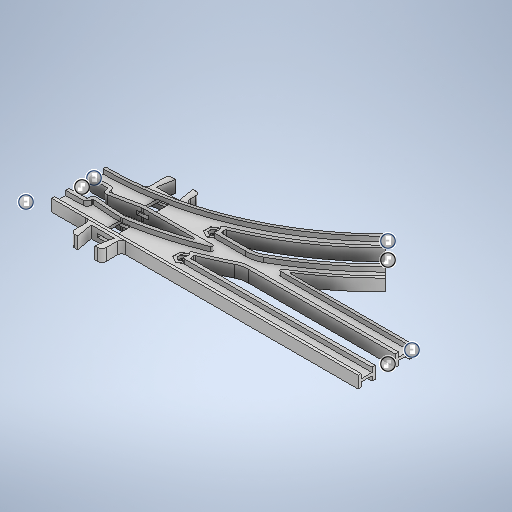
# Autodesk Inventor part: RR_SingleTurnout-all
Saved by Autodesk Inventor 2025.1 (Build 291241000, 241)
## iProperties
Created: 2025-03-05
Part Number: RR_SingleTurnout-all
Material: 一般
Document SubType Name: Modeling
Designer: kumagai
Density: 1 g/cm^3
Appearance: 既定
d0: 244.000 mm
d1: 10.000 mm
d2: 215.000 mm
d3: 5.000 mm
d4: 38.000 mm
d5: 18.600 mm
d6: 2.000 mm
d7: 2.400 mm
d8: 215.000 mm
d9: 45.00 deg
d11: 15.000 mm
d12: 15.000 mm
d13: 2.000 mm
d14: 0.00 deg
d15: 8.400 mm
d16: 0.00 deg
d17: 0.500 mm
d18: 1.000 mm
d19: 20.000 mm
d20: 20.000 mm
d21: 0.500 mm
d22: 1.000 mm
d23: 3.000 mm
d26: 3.000 mm
d27: 3.500 mm
d28: 2.400 mm
d29: 1.000 mm
d30: 5.000 mm
d32: 3.000 mm
d33: 3.000 mm
d34: 3.500 mm
d35: 2.400 mm
d36: 3.000 mm
d37: 1.000 mm
d38: 5.000 mm
d39: 19.000 mm
d41: 0.000 mm
d42: 0.000 mm
d43: 0.000 mm
d44: 0.000 mm
d45: 0.000 mm
d46: 0.000 mm
d47: 0.000 mm
d48: 0.000 mm
d49: 0.000 mm
d51: 6.000 mm
d52: 10.700 mm
d53: 0.300 mm
d55: 2.400 mm
d56: 10.000 mm
d57: 6.000 mm
d58: 0.300 mm
d59: 2.000 mm
d60: 5.000 mm
d62: 2.400 mm
d63: 1.200 mm
d65: 1.200 mm
d66: 41.500 mm
d67: 36.900 mm
TurnoutRadius: 215.000 mm
d40: 19.000 mm
d50: 10.700 mm
PrinterOffset: 0.000 mm
StraightLength: 215.000 mm
RailWidth: 38.000 mm
OuterWall: 2.000 mm
InnerWall: 2.400 mm
InsideWidth: 18.600 mm
RailHeight: 8.400 mm
RailDepth: 3.200 mm
ConnectorLength: 15.000 mm
JointMW1: 13.000 mm
JointMW2: 9.400 mm
JointMH: 9.000 mm
JointFW1: 13.300 mm
JointFW2: 9.600 mm
JointFH: 9.500 mm
DoubleWidth: 60.000 mm
ViaductHeight: 66.000 mm
SupportGap: 0.200 mm
SupportRib: 0.650 mm
JointRadius: 12.000 mm
JointRSLength: 15.000 mm
JointRSTP: 3.000 mm
RailThick: 2.000 mm
Author: kumagai
Autodesk Inventor part; units mm, degrees
ref_plane "YZ Plane" through (0, 0, 0) normal (1, 0, 0) x (0, 1, 0)
ref_plane "XY Plane" through (0, 0, 0) normal (0, 0, 1) x (1, 0, 0)
sketch "MainSketch" plane through (0, 0, 0) normal (0, 1, 0) x (-1, 0, 0)
  line L0 (0, -306.5136) -> (0, 56.9483) projected
  line L1 (-275.3685, 0) -> (77.2109, 0) projected
  line L2 (14.6359, -29) -> (-5, -29)
  line L3 (-5, -49.5106) -> (-5, -5.6416)
  line L4 (-5, -48) -> (0, -48)
  line L5 (-5, -10) -> (0, -10)
  line L6 (-5, -38.3) -> (0, -38.3)
  line L7 (-5, -19.7) -> (0, -19.7)
  line L8 (-5, -46) -> (0, -46)
  line L9 (-5, -35.9) -> (0, -35.9)
  line L10 (-5, -22.1) -> (0, -22.1)
  line L11 (-5, -12) -> (0, -12)
  line L12 (-10, -10) -> (-225, -10)
  line L13 (-10, -10) -> (-10, -48)
  line L14 (-225, -48) -> (-225, -10)
  line L15 (-10, -12) -> (-225, -12)
  line L16 (-93.0964, -19.7) -> (-225, -19.7)
  arc A0 (-10, -48) -> (-148.5929, -105.4071) centre (-10, -244) ccw
  arc A1 (-10, -46) -> (-150.0071, -103.9929) centre (-10, -244) ccw
  line L17 (-143.2215, -110.7785) -> (-189.5102, -64.4898)
  line L18 (-210, -35.9) -> (-210, -22.1)
  line L19 (-146.1596, -86.6272) -> (-155.9415, -76.8453)
  arc A2 (-133.8847, -47.8455) -> (-174.0488, -79.9512) centre (-10, -244) ccw
  arc A3 (-139.2229, -48.9168) -> (-175.463, -78.537) centre (-10, -244) ccw
  line L20 (-139.499, -48) -> (-225, -48)
  line L21 (-134.4186, -46) -> (-225, -46)
  arc A4 (-118.9103, -50.6657) -> (-166.907, -87.093) centre (-10, -244) ccw
  arc A5 (-120.0882, -48.5746) -> (-168.6041, -85.3959) centre (-10, -244) ccw
  line L22 (-88.3997, -46) -> (-110.2721, -46)
  arc A6 (-91.8079, -26.9022) -> (-113.1913, -36.2127) centre (-10, -244) ccw
  line L23 (-122.0871, -35.9) -> (-225, -35.9)
  line L24 (-122.0871, -38.3) -> (-225, -38.3)
  arc A7 (-133.8847, -47.8455) -> (-134.4186, -46) centre (-134.4186, -47) ccw
  arc A8 (-139.2229, -48.9168) -> (-139.499, -48) centre (-139.499, -48.5) ccw
  arc A9 (-110.2721, -48.4) -> (-118.9103, -50.6657) centre (-110.2721, -66) ccw
  arc A10 (-110.2721, -46) -> (-120.0882, -48.5746) centre (-110.2721, -66) ccw
  arc A11 (-122.0871, -38.3) -> (-113.1913, -36.2127) centre (-122.0871, -18.3) ccw
  arc A12 (-122.0871, -35.9) -> (-114.2588, -34.0632) centre (-122.0871, -18.3) ccw
  arc A13 (-84.3565, -34.9289) -> (-84.1889, -35.9) centre (-84.1889, -35.4) ccw
  arc A14 (-94.865, -36.3743) -> (-94.4867, -38.3) centre (-94.4867, -37.3) ccw
  arc A15 (-103.9259, -28.5866) -> (-108.3051, -30.5495) centre (-10, -244) ccw
  arc A16 (-92.2005, -21.1444) -> (-91.4727, -25.2405) centre (-89.0652, -22.7) ccw
  arc A17 (-95.2936, -25.6691) -> (-114.2588, -34.0632) centre (-10, -244) ccw
  line L25 (-95.9536, -22.1) -> (-225, -22.1)
  arc A18 (-94.9553, -23.042) -> (-94.7021, -24.4424) centre (-89.0652, -22.7) ccw
  arc A19 (-91.8079, -26.9022) -> (-91.4727, -25.2405) centre (-92.1605, -25.9664) ccw
  arc A20 (-92.2005, -21.1444) -> (-93.0964, -19.7) centre (-93.0964, -20.7) ccw
  arc A21 (-95.2936, -25.6691) -> (-94.7021, -24.4424) centre (-95.6575, -24.7377) ccw
  arc A22 (-94.9553, -23.042) -> (-95.9536, -22.1) centre (-95.9536, -23.1) ccw
  circle A23 centre (-89.0652, -22.7) radius 2.5
  arc A24 (-96.0029, -53.8443) -> (-104.887, -58.1179) centre (-10, -244) ccw
  arc A25 (-90.2587, -49.342) -> (-89.9638, -50.8719) centre (-84.3686, -49) ccw
  arc A26 (-87.5039, -47.4444) -> (-86.7188, -51.5936) centre (-84.3686, -49) ccw
  arc A27 (-90.5252, -52.1112) -> (-157.1489, -96.8511) centre (-10, -244) ccw
  line L26 (-91.257, -48.4) -> (-110.2721, -48.4)
  arc A28 (-87.0159, -53.2618) -> (-155.4519, -98.5481) centre (-10, -244) ccw
  arc A29 (-87.0159, -53.2618) -> (-86.7188, -51.5936) centre (-87.3903, -52.3346) ccw
  arc A30 (-87.5039, -47.4444) -> (-88.3997, -46) centre (-88.3997, -47) ccw
  arc A31 (-90.5252, -52.1112) -> (-89.9638, -50.8719) centre (-90.9121, -51.1891) ccw
  arc A32 (-90.2587, -49.342) -> (-91.257, -48.4) centre (-91.257, -49.4) ccw
  circle A33 centre (-84.3686, -49) radius 2.5
  line L27 (-43.4568, -12) -> (-26.6853, -12)
  arc A34 (-26.6638, -12.5992) -> (-88.0559, -25.5251) centre (-10, -244) ccw
  arc A35 (-89.0652, -19.7) -> (-88.0559, -25.5251) centre (-89.0652, -22.7) ccw
  arc A36 (-26.6638, -12.5992) -> (-26.6853, -12) centre (-26.6853, -12.3) ccw
  arc A37 (-43.4568, -12) -> (-76.6882, -19.2867) centre (-10, -244) ccw
  line L28 (-89.0652, -19.7) -> (-79.5332, -19.7)
  arc A38 (-79.5332, -19.7) -> (-76.6882, -19.2867) centre (-79.5332, -9.7) ccw
  circle A39 centre (-84.3686, -49) radius 3
  line L29 (-84.9577, -46.0584) -> (-27.1511, -34.4821)
  arc A40 (-27.0106, -35.065) -> (-41.7023, -39.8438) centre (26.8424, -225.6007) ccw
  arc A41 (-27.0106, -35.065) -> (-27.1511, -34.4821) centre (-27.0922, -34.7763) ccw
  arc A42 (-74.694, -46.7073) -> (-82.77, -51.5386) centre (26.8424, -225.6007) ccw
  line L30 (-73.2077, -46.153) -> (-41.7023, -39.8438)
  arc A43 (-73.2077, -46.153) -> (-74.694, -46.7073) centre (-72.2259, -51.0557) ccw
  arc A44 (-48.4878, -13.998) -> (-81.6596, -22.083) centre (-10, -244) ccw
  arc A45 (-27.9859, -39.0878) -> (-44.4613, -41.2072) centre (-10, -244) ccw
  line L31 (-33.0916, -19.7) -> (-48.0227, -19.7)
  line L32 (-25.8398, -35.9879) -> (-26.1688, -34.3986)
  line L33 (-26.7598, -34.0104) -> (-46.4779, -38.0924)
  line L34 (-46.9644, -35.7422) -> (-27.2463, -31.6602)
  line L35 (-23.8186, -33.9121) -> (-23.4896, -35.5014)
  line L36 (-10, -38.3) -> (-23, -38.3)
  line L37 (-48.5051, -38.3) -> (-94.4867, -38.3)
  line L38 (-10, -35.9) -> (-23, -35.9)
  line L39 (-48.5051, -35.9) -> (-84.1889, -35.9)
  arc A46 (-25.8398, -35.9879) -> (-23, -38.3) centre (-23, -35.4) ccw
  arc A47 (-23.4896, -35.5014) -> (-23, -35.9) centre (-23, -35.4) ccw
  arc A48 (-23.8186, -33.9121) -> (-27.2463, -31.6602) centre (-26.6584, -34.5) ccw
  arc A49 (-26.1688, -34.3986) -> (-26.7598, -34.0104) centre (-26.6584, -34.5) ccw
  arc A50 (-48.5051, -38.3) -> (-46.4779, -38.0924) centre (-48.5051, -28.3) ccw
  arc A51 (-48.5051, -35.9) -> (-46.9644, -35.7422) centre (-48.5051, -28.3) ccw
  arc A52 (-10, -22.1) -> (-22.0271, -22.4262) centre (-10, -244) ccw
  arc A53 (-46.742, -25.163) -> (-84.3565, -34.9289) centre (-10, -244) ccw
  arc A54 (-10, -19.7) -> (-22.1572, -20.0297) centre (-10, -244) ccw
  arc A55 (-47.1394, -22.7961) -> (-94.865, -36.3743) centre (-10, -244) ccw
  arc A56 (-25.455, -23.997) -> (-45.2368, -22.6611) centre (-50.9626, -254.5905) ccw
  line L40 (-24.9, -22.9254) -> (-24.9, -23.5)
  arc A57 (-25.455, -23.997) -> (-24.9, -23.5) centre (-25.4, -23.5) ccw
  arc A58 (-22.1572, -20.0297) -> (-24.9, -22.9254) centre (-22, -22.9254) ccw
  arc A59 (-45.2368, -22.6611) -> (-47.1394, -22.7961) centre (-45.4836, -32.6581) ccw
  arc A60 (-25.7188, -26.3824) -> (-45.296, -25.0604) centre (-50.9626, -254.5905) ccw
  arc A61 (-22.0271, -22.4262) -> (-22.5, -22.9254) centre (-22, -22.9254) ccw
  line L41 (-22.5, -22.9254) -> (-22.5, -23.5)
  arc A62 (-25.7188, -26.3824) -> (-22.5, -23.5) centre (-25.4, -23.5) ccw
  arc A63 (-45.296, -25.0604) -> (-46.742, -25.163) centre (-45.4836, -32.6581) ccw
  line L42 (-51.7, -52.4873) -> (-51.7, -10)
  line L43 (-44.3, -51.0246) -> (-44.3, -10)
  line L44 (-48, 3.3517) -> (-48, 5.0252)
  line L45 (-59, -53) -> (-37, -53)
  line L46 (-59, -8.2) -> (-37, -8.2)
  line L47 (-37, -8.2) -> (-37, 0.8)
  line L48 (-40, 3.8) -> (-42, 3.8)
  line L49 (-42, 3.8) -> (-40, -7.7)
  line L50 (-40, -7.7) -> (-56, -7.7)
  line L51 (-56, -7.7) -> (-54, 3.8)
  line L52 (-54, 3.8) -> (-56, 3.8)
  line L53 (-59, 0.8) -> (-59, -8.2)
  line L54 (-37, -8.2) -> (-37, -10)
  line L55 (-59, -8.2) -> (-59, -10)
  arc A64 (-37, 0.8) -> (-40, 3.8) centre (-40, 0.8) ccw
  arc A65 (-56, 3.8) -> (-59, 0.8) centre (-56, 0.8) ccw
  line L56 (-44.3, -10) -> (-44.3, -7.7)
  line L57 (-51.7, -10) -> (-51.7, -7.7)
  line L58 (-48, -62.1182) -> (-48, -64.3828)
  line L59 (-37, -53) -> (-37, -62)
  line L60 (-40, -65) -> (-42, -65)
  line L61 (-42, -65) -> (-40, -53.5)
  line L62 (-40, -53.5) -> (-56, -53.5)
  line L63 (-56, -53.5) -> (-54, -65)
  line L64 (-54, -65) -> (-56, -65)
  line L65 (-59, -62) -> (-59, -53)
  arc A66 (-40, -65) -> (-37, -62) centre (-40, -62) ccw
  arc A67 (-59, -62) -> (-56, -65) centre (-56, -62) ccw
  line L66 (-37, -53) -> (-37, -49.8686)
  line L67 (-44.3, -51.0246) -> (-44.3, -53.5)
  line L68 (-51.7, -52.4873) -> (-51.7, -53.5)
  arc A68 (-34.3731, -49.5213) -> (-37, -52.498) centre (-34, -52.498) ccw
  arc A69 (-59, -58.1371) -> (-62.8083, -55.2481) centre (-62, -58.1371) ccw
  arc A70 (-37, -7) -> (-34, -10) centre (-34, -7) ccw
  arc A71 (-62, -10) -> (-59, -7) centre (-62, -7) ccw
  point P0 (0, 0)
  point P1 (-90.868, -19.7)
  point P2 (-94.9346, -22.1)
  point P3 (-90.238, -48.4)
  point P4 (-86.1714, -46)
  point P5 (-162.028, -91.972)
  point P6 (-225, -29)
  point P7 (-10, -29)
  point P8 (-48.5835, -39.998)
  point P9 (-47.3213, -38.2297)
  point P10 (-44.3, -25.0872)
  point P11 (-51.7, -26.0534)
  point P12 (-51.7, -39.3983)
  point P13 (-44.3, -37.9164)
  point P14 (-48, 2.002)
  point P15 (-48, -55.998)
  point P16 (-37, 3.8)
  point P17 (-59, 3.8)
  point P18 (-37, -65)
  point P19 (-59, -65)
  point P20 (-59, -54.2238)
  dimension "d3" = 5
  dimension "d8" = 215
  dimension "d9" = 45
  dimension "JointRSLength" = 15
  dimension "d0" = 244
  dimension "d1" = 10
  dimension "d2" = 215
  dimension "d4" = 38
  dimension "d5" = 18.6
  dimension "d6" = 2
  dimension "d7" = 2.4
  dimension "d11" = 15
  dimension "d12" = 15
  dimension "d17" = 0.5
  dimension "d18" = 1
  dimension "d19" = 20
  dimension "d20" = 20
  dimension "d21" = 0.5
  dimension "d22" = 1
  dimension "d23" = 3
  dimension "d26" = 3
  dimension "d27" = 3.5
  dimension "d28" = 2.4
  dimension "d29" = 1
  dimension "d30" = 5
  dimension "d32" = 3
  dimension "d34" = 3.5
  dimension "d35" = 2.4
  dimension "d36" = 3
  dimension "d37" = 1
  dimension "d38" = 5
  dimension "d39" = 19
  dimension "d40" = 19
  dimension "d50" = 10.7
  dimension "d51" = 6
  dimension "d52" = 10.7
  dimension "d53" = 0.3
  dimension "d55" = 2.4
  dimension "d56" = 10
  dimension "d57" = 6
  dimension "d58" = 0.3
  dimension "d60" = 5
  dimension "d62" = 2.4
  dimension "d63" = 1.2
  dimension "d65" = 1.2
  dimension "d66" = 41.5
  dimension "d67" = 36.9
  dimension "d70" = 10
  dimension "d72" = 0.5
  dimension "d73" = 3.8
  dimension "d74" = 0.5
  dimension "d75" = 13
  dimension "d76" = 0.5
  dimension "d78" = 12
  dimension "d79" = 10
  dimension "d80" = 3.8
  dimension "d81" = 0.5
  dimension "d99" = 38.5835
  dimension "d100" = 38.4878
  dimension "d101" = 26
  dimension "d102" = 38
  dimension "d103" = 3.7
  dimension "d104" = 3.7
  dimension "d105" = 3.998
  dimension "d122" = 20.8
  dimension "d123" = 16
  dimension "d124" = 16
  dimension "d125" = 24
  constraints: 153 point on circle, 127 end point, 104 tangent, 72 centre point, 36 point on line, 31 coincident, 22 collinear, 15 equal radius, 13 horizontal, 8 symmetric about line, 6 parallel, 4 vertical, 2 perpendicular, 61 other
  measures "d0" distance from line of L1 point (-10, -244)
  measures "d2" distance from line of L2 point (-10, -244)
  measures "d4" distance between parallel lines of L5 L4
  measures "d5" distance between parallel lines of L7 L6
  measures "d6" distance between parallel lines of L8 L4
  measures "d7" distance between parallel lines of L9 L6
  measures "d17" radius of A8
  measures "d18" radius of A7
  measures "d19" radius of A10
  measures "d20" radius of A11
  measures "d21" radius of A13
  measures "d22" radius of A14
  measures "d23" distance from line of point (-89.065, -22.7) L16
  measures "d26" radial gap between concentric circles of A6 A15
  measures "d27" radius of A16
  measures "d28" radial gap between concentric circles of A18 A16
  measures "d29" radius of A19
  measures "d30" diameter of A23
  measures "d32" distance from line of L22 point (-84.369, -49)
  measures "d34" radius of A26
  measures "d35" radial gap between concentric circles of A25 A26
  measures "d36" radial gap between concentric circles of A24 A28
  measures "d37" radius of A29
  measures "d38" diameter of A33
  measures "d39" distance of point (-162.028, -91.972) A0.end
  measures "d40" distance of A3.end point (-162.028, -91.972)
  measures "d50" distance from line of L15 point (-89.065, -22.7)
  measures "d51" diameter of A35
  measures "d52" distance from line of point (-89.065, -22.7) L27
  measures "d53" radius of A36
  measures "d55" radial gap between concentric circles of A37 A34
  measures "d56" radius of A38
  measures "d57" diameter of A39
  measures "d58" radius of A41
  measures "d60" radius of A43
  measures "d62" distance between parallel lines of L29 L30
  measures "d63" distance from line of point (-48.584, -39.998) L29
  measures "d65" radial gap between concentric circles of A34 A44
  measures "d66" distance of point (-89.065, -22.7) A44.start
  measures "d67" distance of point (-84.369, -49) point (-48.584, -39.998)
  measures "d70" radius of A50
  measures "d72" radius of A49
  measures "d73" distance from line of L36 A48.centre
  measures "d74" radius of A47
  measures "d76" radius of A57
  measures "d79" radius of A59
  measures "d80" vertical distance of A54.start A57.centre
  measures "d81" radius of A61
  measures "d101" vertical distance of A44.start point (-48.584, -39.998)
  measures "d103" distance between parallel lines of L43 L44
  measures "d104" distance between parallel lines of L42 L44
  measures "d105" distance from line of L12 A44.start
  measures "d122" distance between parallel lines of L46 L2
  measures "d123" vertical distance of point (-48, 2.002) A44.start
  measures "d124" vertical distance of point (-48, -55.998) point (-48.584, -39.998)
  measures "d125" distance between parallel lines of L2 L45
extrude "BodyPlate" add sketch "MainSketch" along normal mid plane 2 contours L12 L13 L15 L43 | L43 L15 L42 L12 | L13 A54 A58 L40 A57 A56 L43 A34 A36 L15 | L12 L42 L15 L14 | L43 A37 L42 L15 | L15 A37 L43 | L13 A52 A61 L41 A62 A60 L43 A56 A57 L40 A58 A54 | A36 A34 L43 A37 L15 | L42 A37 A38 L28 A35 A34 A55 A14 L37 L29 A39 A42 A43 L30 A1 L17 A28 A29 A26 A30 L22 A10 A5 A2 A7 L21 L14 L24 A11 A6 A19 A16 A20 L16 L15 | L43 A34 L42 A37 | L42 A34 A35 L28 A38 A37 | L43 A56 A59 A55 L42 A34 | L13 L36 A46 L32 A49 L33 L43 L34 A48 L35 A47 L38 | L16 A20 A16 A19 A6 A11 L24 L14 L23 A12 A17 A21 A18 A22 L25 | L13 A1 L43 L30 A40 A41 L29 L33 A49 L32 A46 L36 | L42 A53 A13 L39 L37 A14 A55 | A55 A59 A56 L43 A60 A63 A53 L42 | A1 L42 L30 L43 | L39 A51 L34 L43 L33 A50 L37 L42 | L21 A7 A2 L17 A3 A8 L20 L14 | L37 A50 L33 L43 L29 L42 | L42 L29 L43 L30 | L30 A43 A42 A39 L29 L42 | L43 L29 A41 A40 L30 | L17 A27 A31 A25 A32 L26 A9 A4 A5 A10 L22 A30 A26 A29 A28 | A39
extrude "BodyWall" add sketch "MainSketch" along normal mid plane 8.4 contours L12 L13 L15 L43 | L43 L15 L42 L12 | L12 L42 L15 L14 | L13 A52 A61 L41 A62 A60 L43 A56 A57 L40 A58 A54 | L13 L36 A46 L32 A49 L33 L43 L34 A48 L35 A47 L38 | L16 A20 A16 A19 A6 A11 L24 L14 L23 A12 A17 A21 A18 A22 L25 | L42 A53 A13 L39 L37 A14 A55 | A55 A59 A56 L43 A60 A63 A53 L42 | L13 A0 L43 A1 | L43 A0 L42 A1 | L39 A51 L34 L43 L33 A50 L37 L42 | L42 A0 L45 L65 L17 A1 | L21 A7 A2 L17 A3 A8 L20 L14 | L17 A27 A31 A25 A32 L26 A9 A4 A5 A10 L22 A30 A26 A29 A28 | A0 L65 L45
extrude "SlideChannel" cut sketch "MainSketch" along normal blind 1.4 and the other way blind 1.2 contours L43 L15 L42 L12 | L43 A37 L42 L15 | L43 A34 L42 A37 | L43 A56 A59 A55 L42 A34 | A55 A59 A56 L43 A60 A63 A53 L42 | A53 A63 A60 L43 L34 A51 L39 L42 | L43 A0 L42 A1 | A1 L42 L30 L43 | L39 A51 L34 L43 L33 A50 L37 L42 | L37 A50 L33 L43 L29 L42 | L42 L29 L43 L30
sketch "SupportSketch" plane through (0, 0, 0) normal (0, 1, 0) x (-1, 0, 0)
  circle A0 centre (-84.3686, -49) radius 2.5 projected
  circle A1 centre (-89.0652, -22.7) radius 2.5 projected
  line L0 (-84.3686, -55.5) -> (-84.3686, -49)
  line L1 (-84.3686, -42.5) -> (-78.7394, -45.75)
  line L2 (-78.7394, -45.75) -> (-84.3686, -49)
  line L3 (-84.3686, -49) -> (-78.7394, -52.25)
  line L4 (-78.7394, -52.25) -> (-84.3686, -55.5)
  line L5 (-89.0652, -29.2) -> (-89.0652, -22.7)
  line L6 (-89.0652, -16.2) -> (-83.4361, -19.45)
  line L7 (-83.4361, -19.45) -> (-89.0652, -22.7)
  line L8 (-89.0652, -22.7) -> (-83.4361, -25.95)
  line L9 (-83.4361, -25.95) -> (-89.0652, -29.2)
  line L10 (-84.3686, -49) -> (-84.3686, -42.5)
  line L11 (-89.0652, -22.7) -> (-89.0652, -16.2)
  line L12 (-83.7186, -54.3742) -> (-83.7186, -50.1258)
  line L13 (-83.7186, -50.1258) -> (-80.0394, -52.25)
  line L14 (-80.0394, -52.25) -> (-83.7186, -54.3742)
  line L15 (-83.7186, -47.8742) -> (-80.0394, -45.75)
  line L16 (-80.0394, -45.75) -> (-83.7186, -43.6258)
  line L17 (-83.7186, -43.6258) -> (-83.7186, -47.8742)
  line L18 (-88.4152, -28.0742) -> (-88.4152, -23.8258)
  line L19 (-88.4152, -23.8258) -> (-84.7361, -25.95)
  line L20 (-84.7361, -25.95) -> (-88.4152, -28.0742)
  line L21 (-88.4152, -21.5742) -> (-84.7361, -19.45)
  line L22 (-84.7361, -19.45) -> (-88.4152, -17.3258)
  line L23 (-88.4152, -17.3258) -> (-88.4152, -21.5742)
  line L24 (-84.3686, -54) -> (-88.6987, -51.5)
  line L25 (-88.6987, -51.5) -> (-88.6987, -46.5)
  line L26 (-88.6987, -46.5) -> (-84.3686, -44)
  line L27 (-84.3686, -44) -> (-80.0385, -46.5)
  line L28 (-80.0385, -46.5) -> (-80.0385, -51.5)
  line L29 (-80.0385, -51.5) -> (-84.3686, -54)
  line L30 (-89.0652, -27.7) -> (-93.3954, -25.2)
  line L31 (-93.3954, -25.2) -> (-93.3954, -20.2)
  line L32 (-93.3954, -20.2) -> (-89.0652, -17.7)
  line L33 (-89.0652, -17.7) -> (-84.7351, -20.2)
  line L34 (-84.7351, -20.2) -> (-84.7351, -25.2)
  line L35 (-84.7351, -25.2) -> (-89.0652, -27.7)
  line L36 (-84.3686, -51.85) -> (-86.8368, -50.425)
  line L37 (-86.8368, -50.425) -> (-86.8368, -47.575)
  line L38 (-86.8368, -47.575) -> (-84.3686, -46.15)
  line L39 (-84.3686, -46.15) -> (-81.9004, -47.575)
  line L40 (-81.9004, -47.575) -> (-81.9004, -50.425)
  line L41 (-81.9004, -50.425) -> (-84.3686, -51.85)
  line L42 (-89.0652, -25.55) -> (-91.5334, -24.125)
  line L43 (-91.5334, -24.125) -> (-91.5334, -21.275)
  line L44 (-91.5334, -21.275) -> (-89.0652, -19.85)
  line L45 (-89.0652, -19.85) -> (-86.5971, -21.275)
  line L46 (-86.5971, -21.275) -> (-86.5971, -24.125)
  line L47 (-86.5971, -24.125) -> (-89.0652, -25.55)
  point P0 (0, 0)
  point P1 (-86.5971, -22.3024)
  point P2 (-86.5971, -23.0976)
  point P3 (-87.4868, -24.6387)
  point P4 (-88.1755, -25.0363)
  point P5 (-89.9549, -25.0363)
  point P6 (-90.6437, -24.6387)
  point P7 (-91.5334, -23.0976)
  point P8 (-91.5334, -22.3024)
  point P9 (-90.6437, -20.7613)
  point P10 (-89.9549, -20.3637)
  point P11 (-88.1755, -20.3637)
  point P12 (-87.4868, -20.7613)
  point P13 (-82.7901, -50.9387)
  point P14 (-83.4789, -51.3363)
  point P15 (-85.2583, -51.3363)
  point P16 (-85.9471, -50.9387)
  point P17 (-86.8368, -49.3976)
  point P18 (-86.8368, -48.6024)
  point P19 (-85.9471, -47.0613)
  point P20 (-85.2583, -46.6637)
  point P21 (-83.4789, -46.6637)
  point P22 (-82.7901, -47.0613)
  point P23 (-81.9004, -48.6024)
  point P24 (-81.9004, -49.3976)
  dimension "d113" = 0.65
  dimension "d114" = 0.65
  dimension "d115" = 0.65
  dimension "d116" = 0.65
  dimension "d117" = 6.5
  dimension "d150" = 5
  dimension "d151" = 2.85
  dimension "d153" = 5
  dimension "d154" = 2.85
  constraints: 96 end point, 11 equal length, 8 coincident, 4 point on line, 2 collinear, 2 vertical, 60 other
  measures "d113" distance between parallel lines of L4 L14
  measures "d114" distance between parallel lines of L1 L16
  measures "d115" distance between parallel lines of L9 L20
  measures "d116" distance between parallel lines of L7 L21
  measures "d117" distance of L3.end L0.start
  measures "d150" distance of L24.end L25.end
  measures "d151" distance of L36.end L37.end
  measures "d153" distance of L30.end L31.end
  measures "d154" distance of L42.end L43.end
ref_plane "SupportTopSurface" through (0, -1.4, 0) normal (0, 1, 0) x (-1, 0, 0)
ref_plane "SupportMidSurface" through (0, -2, 0) normal (0, 1, 0) x (-1, 0, 0)
extrude "Ring" add sketch "SupportSketch" along normal mid plane 2.4 contours A0 L40 L2 L28 L3 | L39 L15 L27 L2 | L3 L29 L13 L41 | L39 A0 L17 L27 L15 | L13 L29 L12 L41 A0 | L36 L0 L24 L25 L26 L10 L38 A0 L37 | L41 L12 L29 L0 | L10 L27 L17 L39 | A1 L46 L7 L34 L8 | L45 L21 L33 L7 | L8 L35 L19 L47 | L45 A1 L23 L33 L21 | L19 L35 L18 L47 A1 | L42 L5 L30 L31 L32 L11 L44 A1 L43 | L47 L18 L35 L5 | L11 L33 L23 L45
ref_plane "BaseSurface" through (0, -4.2, 0) normal (0, 1, 0) x (-1, 0, 0)
extrude "SupportA" add sketch "SupportSketch" along normal up to surface (0.6 mm away) from surface at -2 separate body contours L2 L10 A0 L17 L15 | A0 L15 L39 L2 | L39 L15 L27 L2 | L3 L41 L13 A0 | A0 L13 L12 L0 L3 | L3 L29 L13 L41 | L27 L15 L16 L17 L10 L1 L2 | L3 L4 L0 L29 L12 L14 L13 | A0 L12 L41 L0 | L10 L39 L17 A0 | L41 L12 L29 L0 | L10 L27 L17 L39 | L7 L11 A1 L23 L21 | A1 L21 L45 L7 | L45 L21 L33 L7 | L8 L47 L19 A1 | A1 L19 L18 L5 L8 | L8 L35 L19 L47 | L33 L21 L22 L23 L11 L6 L7 | L8 L9 L5 L35 L18 L20 L19 | A1 L18 L47 L5 | L11 L45 L23 A1 | L47 L18 L35 L5 | L11 L33 L23 L45
extrude "SupportB" add sketch "SupportSketch" against normal up to surface (2.2 mm away) from surface at -2 contours L2 L10 A0 L17 L15 | A0 L15 L39 L2 | L39 L15 L27 L2 | L3 L41 L13 A0 | A0 L13 L12 L0 L3 | L3 L29 L13 L41 | L15 L17 A0 L39 | A0 L39 L15 | L27 L15 L16 L17 L10 L1 L2 | L39 A0 L17 L27 L15 | L13 L41 A0 | A0 L41 L12 L13 | L3 L4 L0 L29 L12 L14 L13 | L13 L29 L12 L41 A0 | L39 A0 | A0 L12 L41 L0 | L10 L39 L17 A0 | L27 L17 L16 L15 | A0 L41 | L13 L14 L12 L29 | A0 L17 L39 | A0 L41 L12 | L41 L12 L29 L0 | L10 L27 L17 L39 | L7 L11 A1 L23 L21 | A1 L21 L45 L7 | L45 L21 L33 L7 | L8 L47 L19 A1 | A1 L19 L18 L5 L8 | L8 L35 L19 L47 | L21 L23 A1 L45 | A1 L45 L21 | L33 L21 L22 L23 L11 L6 L7 | L45 A1 L23 L33 L21 | L19 L47 A1 | A1 L47 L18 L19 | L8 L9 L5 L35 L18 L20 L19 | L19 L35 L18 L47 A1 | L45 A1 | A1 L18 L47 L5 | L11 L45 L23 A1 | L33 L23 L22 L21 | A1 L47 | L19 L20 L18 L35 | A1 L23 L45 | A1 L47 L18 | L47 L18 L35 L5 | L11 L33 L23 L45 bodies 2
extrude "SwitchA" add sketch "MainSketch" along normal mid plane 8.4 separate body contours L47 L46 L56 L50 L49 L1 | L1 L49 L48 A64 L47 | A70 L12 L54 L47 | L51 L50 L57 L46 L53 L1 | L1 L53 A65 L52 L51 | L54 L12 L56 L46 | L56 L46 L57 L50 | L56 L12 L57 L46 | L53 L55 L12 A71 | L57 L12 L55 L46 | A68 L66 A0 | L67 L45 L68 A0 | A0 L66 L45 L67 | L68 L45 A0 | L67 L62 L68 L45 | L45 L59 A66 L60 L61 L62 L67 | L45 L68 L62 L63 L64 A67 L65 A0 | A0 L65 A69
extrude "SwitchB" cut sketch "MainSketch" along normal mid plane 2.4 contours L56 L46 L57 L50 | L56 L12 L57 L46 | L67 L45 L68 A0 | L67 L62 L68 L45 bodies 3
equation "\"d8\" = StraightLength"
equation "\"d2\" = TurnoutRadius"
equation "\"d4\" = RailWidth"
equation "\"d5\" = InsideWidth"
equation "\"d6\" = OuterWall"
equation "\"d7\" = InnerWall"
equation "\"d11\" = JointRSLength"
equation "\"d12\" = JointRSLength"
equation "\"d13\" = RailThick"
equation "\"d15\" = RailHeight"
equation "\"TurnoutRadius\" = StraightLength"
equation "\"StraightLength\" = 215"
equation "\"RailWidth\" = 38"
equation "\"InsideWidth\" = 18.6"
equation "\"OuterWall\" = 2"
equation "\"InnerWall\" = 2.4"
equation "\"RailThick\" = 2"
equation "\"RailHeight\" = 8.4"
